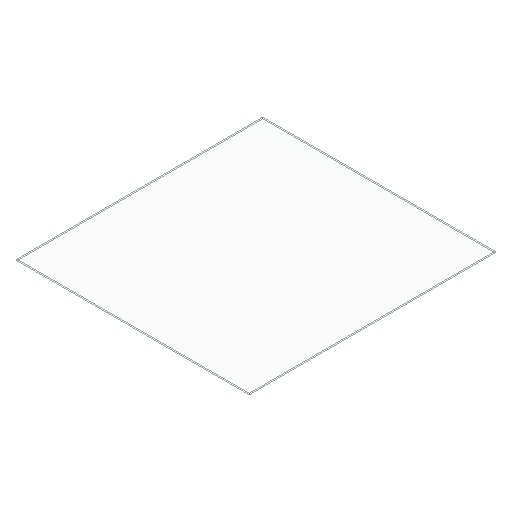
# Autodesk Inventor part: CUT_Heatbed_2mm_Glass
Saved by Autodesk Inventor 2026.1 (Build 301233000, 233)
## iProperties
Created: 2016-06-21
Part Number: CUT_Heatbed_2mm_Glass
Material: Ogólny
Document SubType Name: Modeling
Designer: Andrzej
Density: 1 g/cm^3
Appearance: Szkło pełne
Mass: 788.873 g
Surface Area: 2716.6 cm^2
Volume: 788.873 cm^3
Author: Andrzej
Autodesk Inventor part; units mm, degrees
ref_plane "YZ Plane" through (0, 0, 0) normal (1, 0, 0) x (0, 1, 0)
ref_plane "XZ Plane" through (0, 0, 0) normal (0, 1, 0) x (-1, 0, 0)
ref_plane "XY Plane" through (0, 0, 0) normal (0, 0, 1) x (1, 0, 0)
sketch "Szkic1" plane through (0, 0, 0) normal (0, 0, 1) x (1, 0, 0)
  line L0 (9.4719, 9.8006) -> (352.0719, 9.8006)
  line L1 (352.0719, 9.8006) -> (352.0719, -352.7994)
  line L2 (352.0719, -352.7994) -> (9.4719, -352.7994)
  line L3 (9.4719, -352.7994) -> (9.4719, 9.8006)
  point P0 (0, 0)
  point P1 (24.4719, -337.7994)
  point P2 (337.0719, -337.7994)
  point P3 (24.4719, -5.1994)
  point P4 (337.0719, -5.1994)
  dimension "d0" = 342.6
  dimension "d1" = 362.6
  dimension "d4" = 15
  dimension "d5" = 15
  dimension "d6" = 15
  dimension "d7" = 15
  dimension "d8" = 15
  dimension "d9" = 15
  dimension "d10" = 15
  dimension "d11" = 15
  dimension "d19" = 312.6
  dimension "d20" = 332.6
  constraints: 8 end point, 2 parallel, 1 horizontal, 1 perpendicular
  measures "d0" distance of L1.end L2.end
  measures "d1" distance of L0.end L1.end
  measures "d4" distance from line of point (24.472, -337.799) L2
  measures "d5" distance from line of point (24.472, -337.799) L3
  measures "d6" distance from line of L2 point (337.072, -337.799)
  measures "d7" distance from line of L1 point (337.072, -337.799)
  measures "d8" distance from line of L1 point (337.072, -5.199)
  measures "d9" distance from line of L0 point (337.072, -5.199)
  measures "d10" distance from line of L3 point (24.472, -5.199)
  measures "d11" distance from line of L0 point (24.472, -5.199)
  measures "d19" distance of point (24.472, -5.199) point (337.072, -5.199)
  measures "d20" distance of point (337.072, -337.799) point (337.072, -5.199)
extrude "Wyciągnięcie proste1" add sketch "Szkic1" along normal blind 2
equation "\"d5\" = d4"
equation "\"d6\" = d4"
equation "\"d7\" = d4"
equation "\"d8\" = d4"
equation "\"d9\" = d4"
equation "\"d10\" = d4"
equation "\"d11\" = d4"
